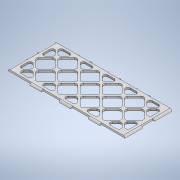
# Autodesk Inventor part: bottom
Saved by Autodesk Inventor 2020 (Build 240168000, 168)
## iProperties
Created: 2020-06-10
Part Number: bottom
Material: Generic
Document SubType Name: Modeling
Designer: maple
Density: 1 g/cm^3
Appearance: Default
Author: maple
Autodesk Inventor part; units mm, degrees
ref_plane "YZ Plane" through (0, 0, 0) normal (1, 0, 0) x (0, 1, 0)
ref_plane "XZ Plane" through (0, 0, 0) normal (0, 1, 0) x (-1, 0, 0)
ref_plane "XY Plane" through (0, 0, 0) normal (0, 0, 1) x (1, 0, 0)
sketch "Sketch1" plane through (0, 0, 0) normal (0, 1, 0) x (-1, 0, 0)
  line L0 (0, 0) -> (-100, 0)
  line L1 (-100, 0) -> (-100, -40)
  line L2 (-100, -40) -> (0, -40)
  line L3 (0, -40) -> (0, 0)
  line L4 (0, 0) -> (-25, 0)
  line L5 (-25, 0) -> (-50, 0)
  line L6 (-50, 0) -> (-75, 0)
  line L7 (-75, 0) -> (-100, 0)
  line L8 (-25, 0) -> (-20, 0)
  line L9 (-20, 0) -> (-30, 0)
  line L10 (-30, 0) -> (-30, 1.5)
  line L11 (-30, 1.5) -> (-20, 1.5)
  line L12 (-20, 1.5) -> (-20, 0)
  line L13 (-50, 0) -> (-45, 0)
  line L14 (-45, 0) -> (-55, 0)
  line L15 (-55, 0) -> (-55, 1.5)
  line L16 (-55, 1.5) -> (-45, 1.5)
  line L17 (-45, 1.5) -> (-45, 0)
  line L18 (-75, 0) -> (-70, 0)
  line L19 (-70, 0) -> (-80, 0)
  line L20 (-80, 0) -> (-80, 1.5)
  line L21 (-80, 1.5) -> (-70, 1.5)
  line L22 (-70, 1.5) -> (-70, 0)
  line L23 (-100, -20) -> (-100, -15)
  line L24 (-100, -15) -> (-98.5, -15)
  line L25 (-98.5, -15) -> (-98.5, -25)
  line L26 (-98.5, -25) -> (-100, -25)
  line L27 (-100, -25) -> (-100, -15)
  line L28 (0, -20) -> (0, -15)
  line L29 (0, -15) -> (-1.5, -15)
  line L30 (-1.5, -15) -> (-1.5, -25)
  line L31 (-1.5, -25) -> (0, -25)
  line L32 (0, -25) -> (0, -15)
  line L33 (-20, -40) -> (-30, -40)
  line L34 (-45, -40) -> (-55, -40)
  line L35 (-70, -40) -> (-80, -40)
  line L36 (0, -20) -> (-2.5, -20)
  line L37 (-2.5, -20) -> (-21.5, -20)
  line L38 (-21.5, -20) -> (-40.5, -20)
  line L39 (-40.5, -20) -> (-59.5, -20)
  line L40 (-59.5, -20) -> (-78.5, -20)
  line L41 (-78.5, -20) -> (-97.5, -20)
  line L42 (-97.5, -20) -> (-100, -20)
  line L43 (-2.5, -20) -> (-3.5, -20)
  line L44 (-3.5, -20) -> (-12, -28.5)
  line L45 (-12, -28.5) -> (-20.5, -20)
  line L46 (-20.5, -20) -> (-12, -11.5)
  line L47 (-12, -11.5) -> (-3.5, -20)
  line L48 (-39.5, -20) -> (-31, -11.5)
  line L49 (-31, -11.5) -> (-22.5, -20)
  line L50 (-22.5, -20) -> (-31, -28.5)
  line L51 (-31, -28.5) -> (-39.5, -20)
  line L52 (-58.5, -20) -> (-50, -11.5)
  line L53 (-50, -11.5) -> (-41.5, -20)
  line L54 (-41.5, -20) -> (-50, -28.5)
  line L55 (-50, -28.5) -> (-58.5, -20)
  line L56 (-77.5, -20) -> (-69, -11.5)
  line L57 (-69, -11.5) -> (-60.5, -20)
  line L58 (-60.5, -20) -> (-69, -28.5)
  line L59 (-69, -28.5) -> (-77.5, -20)
  line L60 (-96.5, -20) -> (-88, -11.5)
  line L61 (-88, -11.5) -> (-79.5, -20)
  line L62 (-79.5, -20) -> (-88, -28.5)
  line L63 (-88, -28.5) -> (-96.5, -20)
  line L64 (-13, -10.5) -> (-21.5, -19)
  line L65 (-21.5, -19) -> (-30, -10.5)
  line L66 (-30, -10.5) -> (-21.5, -2)
  line L67 (-21.5, -2) -> (-13, -10.5)
  line L68 (-13, -29.5) -> (-21.5, -38)
  line L69 (-21.5, -38) -> (-30, -29.5)
  line L70 (-30, -29.5) -> (-21.5, -21)
  line L71 (-21.5, -21) -> (-13, -29.5)
  line L72 (-12, -9.5) -> (-19.5, -2)
  line L73 (-12, -9.5) -> (-1.3934, -9.5) construction
  line L74 (-19.5, -2) -> (-4.5, -2)
  line L75 (-4.5, -2) -> (-12, -9.5)
  line L76 (-12, -30.5) -> (-4.5, -38)
  line L77 (-4.5, -38) -> (-19.5, -38)
  line L78 (-19.5, -38) -> (-12, -30.5)
  line L79 (-32, -10.5) -> (-40.5, -19)
  line L80 (-40.5, -2) -> (-32, -10.5)
  line L81 (-49, -10.5) -> (-40.5, -2)
  line L82 (-40.5, -19) -> (-49, -10.5)
  line L83 (-40.5, -21) -> (-32, -29.5)
  line L84 (-49, -29.5) -> (-40.5, -21)
  line L85 (-40.5, -38) -> (-49, -29.5)
  line L86 (-32, -29.5) -> (-40.5, -38)
  line L87 (-51, -10.5) -> (-59.5, -19)
  line L88 (-59.5, -2) -> (-51, -10.5)
  line L89 (-68, -10.5) -> (-59.5, -2)
  line L90 (-59.5, -19) -> (-68, -10.5)
  line L91 (-59.5, -21) -> (-51, -29.5)
  line L92 (-68, -29.5) -> (-59.5, -21)
  line L93 (-59.5, -38) -> (-68, -29.5)
  line L94 (-51, -29.5) -> (-59.5, -38)
  line L95 (-70, -10.5) -> (-78.5, -19)
  line L96 (-78.5, -2) -> (-70, -10.5)
  line L97 (-87, -10.5) -> (-78.5, -2)
  line L98 (-78.5, -19) -> (-87, -10.5)
  line L99 (-78.5, -21) -> (-70, -29.5)
  line L100 (-87, -29.5) -> (-78.5, -21)
  line L101 (-78.5, -38) -> (-87, -29.5)
  line L102 (-70, -29.5) -> (-78.5, -38)
  line L103 (-23.5, -2) -> (-31, -9.5)
  line L104 (-38.5, -2) -> (-23.5, -2)
  line L105 (-31, -9.5) -> (-38.5, -2)
  line L106 (-31, -30.5) -> (-23.5, -38)
  line L107 (-38.5, -38) -> (-31, -30.5)
  line L108 (-23.5, -38) -> (-38.5, -38)
  line L109 (-42.5, -2) -> (-50, -9.5)
  line L110 (-57.5, -2) -> (-42.5, -2)
  line L111 (-50, -9.5) -> (-57.5, -2)
  line L112 (-50, -30.5) -> (-42.5, -38)
  line L113 (-57.5, -38) -> (-50, -30.5)
  line L114 (-42.5, -38) -> (-57.5, -38)
  line L115 (-61.5, -2) -> (-69, -9.5)
  line L116 (-76.5, -2) -> (-61.5, -2)
  line L117 (-69, -9.5) -> (-76.5, -2)
  line L118 (-69, -30.5) -> (-61.5, -38)
  line L119 (-76.5, -38) -> (-69, -30.5)
  line L120 (-61.5, -38) -> (-76.5, -38)
  line L121 (-80.5, -2) -> (-88, -9.5)
  line L122 (-95.5, -2) -> (-80.5, -2)
  line L123 (-88, -9.5) -> (-95.5, -2)
  line L124 (-88, -30.5) -> (-80.5, -38)
  line L125 (-95.5, -38) -> (-88, -30.5)
  line L126 (-80.5, -38) -> (-95.5, -38)
  line L127 (-11, -10.5) -> (-3.5, -18)
  line L128 (-3.5, -18) -> (-3.5, -3)
  line L129 (-3.5, -3) -> (-11, -10.5)
  line L130 (-11, -29.5) -> (-3.5, -22)
  line L131 (-3.5, -22) -> (-3.5, -37)
  line L132 (-3.5, -37) -> (-11, -29.5)
  line L133 (-89, -10.5) -> (-96.5, -18)
  line L134 (-96.5, -18) -> (-96.5, -3)
  line L135 (-96.5, -3) -> (-89, -10.5)
  line L136 (-89, -29.5) -> (-96.5, -37)
  line L137 (-96.5, -37) -> (-96.5, -22)
  line L138 (-96.5, -22) -> (-89, -29.5)
  line L139 (-20, -40) -> (-30, -40)
  line L140 (-30, -40) -> (-30, -41.5)
  line L141 (-30, -41.5) -> (-20, -41.5)
  line L142 (-20, -41.5) -> (-20, -40)
  line L143 (-45, -40) -> (-55, -40)
  line L144 (-55, -40) -> (-55, -41.5)
  line L145 (-55, -41.5) -> (-45, -41.5)
  line L146 (-45, -41.5) -> (-45, -40)
  line L147 (-70, -40) -> (-80, -40)
  line L148 (-80, -40) -> (-80, -41.5)
  line L149 (-80, -41.5) -> (-70, -41.5)
  line L150 (-70, -41.5) -> (-70, -40)
  point P0 (-12, -20)
  point P1 (-21.5, -10.5)
  point P2 (-21.5, -29.5)
  dimension "d0" = 100
  dimension "d1" = 40
  dimension "d2" = 25
  dimension "d3" = 25
  dimension "d4" = 25
  dimension "d5" = 25
  dimension "d6" = 5
  dimension "d7" = 10
  dimension "d8" = 1.5
  dimension "d9" = 5
  dimension "d10" = 10
  dimension "d11" = 1.5
  dimension "d12" = 5
  dimension "d13" = 10
  dimension "d14" = 1.5
  dimension "d15" = 5
  dimension "d16" = 1.5
  dimension "d17" = 10
  dimension "d18" = 5
  dimension "d19" = 1.5
  dimension "d20" = 10
  dimension "d27" = 2.5
  dimension "d28" = 19
  dimension "d29" = 19
  dimension "d30" = 19
  dimension "d31" = 19
  dimension "d32" = 19
  dimension "d33" = 2.5
  dimension "d34" = 1
  dimension "d37" = 19
  dimension "d42" = 135
  dimension "d45" = 19
  dimension "d52" = 19
  dimension "d57" = 10
  dimension "d58" = 1.5
  dimension "d59" = 10
  dimension "d60" = 1.5
  dimension "d61" = 10
  dimension "d62" = 1.5
  constraints: 302 end point, 22 equal length, 19 horizontal, 19 point on line, 18 perpendicular, 4 midpoint, 2 vertical, 155 other
  measures "d0" distance of L2.end L1.end
  measures "d1" distance of L1.end L0.end
  measures "d2" distance of L0.start L4.end
  measures "d3" distance of L4.end L5.end
  measures "d4" distance of L5.end L6.end
  measures "d5" distance of L6.end L0.end
  measures "d6" distance of L4.end L8.end
  measures "d7" distance of L10.end L11.end
  measures "d8" distance of L9.end L10.end
  measures "d9" distance of L5.end L13.end
  measures "d10" distance of L15.end L16.end
  measures "d11" distance of L14.end L15.end
  measures "d12" distance of L6.end L18.end
  measures "d13" distance of L20.end L21.end
  measures "d14" distance of L19.end L20.end
  measures "d15" distance of L23.start L23.end
  measures "d16" distance of L25.end L26.end
  measures "d17" distance of L24.end L25.end
  measures "d18" distance of L28.start L28.end
  measures "d19" distance of L31.end L30.end
  measures "d20" distance of L30.end L29.end
  measures "d27" distance of L28.start L36.end
  measures "d28" distance of L36.end L37.end
  measures "d29" distance of L37.end L38.end
  measures "d30" distance of L38.end L39.end
  measures "d31" distance of L39.end L40.end
  measures "d32" distance of L40.end L41.end
  measures "d33" distance of L41.end L23.start
  measures "d34" distance of L36.end L43.end
  measures "d37" distance of L45.end L48.start
  measures "d42" angle of L73 L72
  measures "d45" distance of L64.start L79.start
  measures "d52" distance of L74.end L103.start
  measures "d57" distance of L141.end L140.end
  measures "d58" distance of L140.end L139.end
  measures "d59" distance of L145.end L144.end
  measures "d60" distance of L144.end L143.end
  measures "d61" distance of L149.end L148.end
  measures "d62" distance of L148.end L147.end
extrude "Extrusion1" add sketch "Sketch1" along normal blind 1.5 contours L3 L29 L30 L36 L37 L47 L46 L38 L49 L48 L39 L53 L52 L40 L57 L56 L41 L61 L60 L42 L25 L24 L1 L0 | L0 L10 L11 L12 | L3 L2 L1 L26 L25 L42 L41 L63 L62 L40 L59 L58 L39 L55 L54 L38 L51 L50 L37 L45 L44 L36 L30 L31 | L0 L15 L16 L17 | L142 L141 L140 L2 | L0 L20 L21 L22 | L146 L145 L144 L2 | L150 L149 L148 L2
fillet "Fillet1" radius 2 94 edges at (4.5, 0.75, -2) (3.5, 0.75, -3) (3.5, 0.75, -22) (3.5, 0.75, -18) (3.5, 0.75, -37) (11, 0.75, -10.5) (11, 0.75, -29.5) (20.5, 0.75, -20) (3.5, 0.75, -20) (13, 0.75, -10.5) (13, 0.75, -29.5) (22.5, 0.75, -20) (30, 0.75, -10.5) (30, 0.75, -29.5) (32, 0.75, -10.5) (39.5, 0.75, -20) (49, 0.75, -10.5) (51, 0.75, -10.5) (49, 0.75, -29.5) (51, 0.75, -29.5) (58.5, 0.75, -20) (60.5, 0.75, -20) (68, 0.75, -29.5) (68, 0.75, -10.5) (70, 0.75, -10.5) (77.5, 0.75, -20) (79.5, 0.75, -20) (70, 0.75, -29.5) (87, 0.75, -10.5) (89, 0.75, -10.5) (96.5, 0.75, -20) (87, 0.75, -29.5) (89, 0.75, -29.5) (41.5, 0.75, -20) (32, 0.75, -29.5) (19.5, 0.75, -2) (38.5, 0.75, -2) (57.5, 0.75, -2) (42.5, 0.75, -2) (61.5, 0.75, -2) (76.5, 0.75, -2) (80.5, 0.75, -2) (95.5, 0.75, -2) (96.5, 0.75, -3) (96.5, 0.75, -18) (95.5, 0.75, -38) (80.5, 0.75, -38) (76.5, 0.75, -38) (61.5, 0.75, -38) (57.5, 0.75, -38) (42.5, 0.75, -38) (38.5, 0.75, -38) (23.5, 0.75, -38) (19.5, 0.75, -38) (4.5, 0.75, -38) (96.5, 0.75, -37) (96.5, 0.75, -22) (12, 0.75, -9.5) (12, 0.75, -11.5) (12, 0.75, -30.5) (12, 0.75, -28.5) (21.5, 0.75, -2) (21.5, 0.75, -19) (21.5, 0.75, -21) (21.5, 0.75, -38) (23.5, 0.75, -2) (31, 0.75, -9.5) (31, 0.75, -11.5) (31, 0.75, -28.5) (31, 0.75, -30.5) (40.5, 0.75, -2) (40.5, 0.75, -19) (40.5, 0.75, -21) (40.5, 0.75, -38) (59.5, 0.75, -2) (50, 0.75, -11.5) (50, 0.75, -9.5) (50, 0.75, -30.5) (50, 0.75, -28.5) (59.5, 0.75, -19) (59.5, 0.75, -21) (59.5, 0.75, -38) (69, 0.75, -9.5) (69, 0.75, -11.5) (69, 0.75, -28.5) (69, 0.75, -30.5) (78.5, 0.75, -2) (78.5, 0.75, -19) (78.5, 0.75, -21) (78.5, 0.75, -38) (88, 0.75, -9.5) (88, 0.75, -11.5) (88, 0.75, -28.5) (88, 0.75, -30.5)
fillet "Fillet2" radius 1.5 10 edges at (25, 1.5, 1.5) (50, 1.5, 1.5) (75, 1.5, 1.5) (75, 1.5, -41.5) (50, 1.5, -41.5) (25, 1.5, -41.5) (0, 1.5, -7.5) (0, 1.5, -32.5) (100, 1.5, -7.5) (100, 1.5, -32.5)
body "Solid1"
